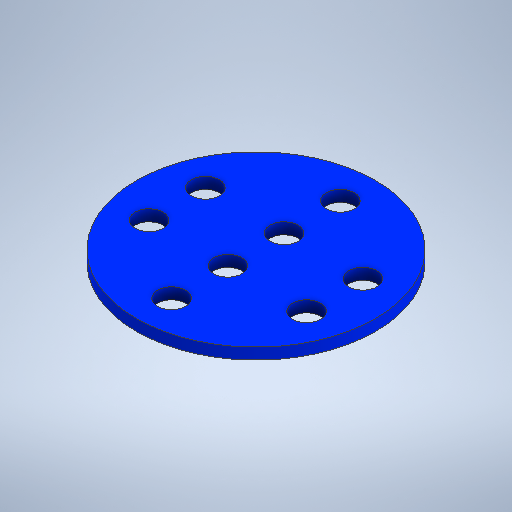
# Autodesk Inventor part: Wires_Base
Saved by Autodesk Inventor 2025.2 (Build 292293000, 293)
## iProperties
Created: 2025-02-12
Part Number: Wires_Base
Material: Generic
Document SubType Name: Modeling
Designer: User
Density: 1 g/cm^3
Appearance: Default
Author: User
Autodesk Inventor part; units mm, degrees
ref_plane "YZ Plane" through (0, 0, 0) normal (1, 0, 0) x (0, 1, 0)
ref_plane "XZ Plane" through (0, 0, 0) normal (0, 1, 0) x (-1, 0, 0)
ref_plane "XY Plane" through (0, 0, 0) normal (0, 0, 1) x (1, 0, 0)
sketch "Sketch1" plane through (0, 0, 0) normal (0, 1, 0) x (-1, 0, 0)
  circle A0 centre (0, 0) radius 42.5
  line L0 (0, 0) -> (0, -5)
  line L1 (0, 0) -> (0, 5)
  circle A1 centre (28, 10) radius 5
  circle A2 centre (0, 10) radius 5
  circle A3 centre (-28, 10) radius 5
  circle A4 centre (28, -10) radius 5
  circle A5 centre (-28, -10) radius 5
  circle A6 centre (0, -10) radius 5
  circle A7 centre (0, 30) radius 5
  circle A8 centre (0, -30) radius 5
  dimension "d2" = 85
  dimension "d5" = 10
  dimension "d6" = 10
  dimension "d7" = 10
  dimension "d10" = 10
  dimension "d11" = 10
  dimension "d12" = 10
  dimension "d13" = 10
  dimension "d15" = 10
  constraints: 9 centre point, 4 end point, 2 vertical, 1 coincident
  measures "d2" diameter of A0
  measures "d5" diameter of A1
  measures "d6" diameter of A2
  measures "d7" diameter of A3
  measures "d10" diameter of A4
  measures "d11" diameter of A5
  measures "d12" diameter of A6
  measures "d13" diameter of A7
  measures "d15" diameter of A8
extrude "Extrusion1" add sketch "Sketch1" along normal blind 4
body "Solid1"
